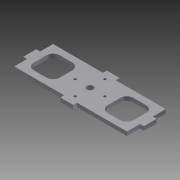
# Autodesk Inventor part: OpenROV 2_2 Horizontal Bulkhead
Saved by Autodesk Inventor 2011 (Build 150239000, 239)
## iProperties
Created: 2011-11-06
Part Number: OpenROV 2_2 Horizontal Bulkhead
Document SubType Name: Modeling
Designer: user
Density: 1 g/cm^3
Author: user
Autodesk Inventor part; units mm, degrees
ref_plane "YZ Plane" through (0, 0, 0) normal (1, 0, 0) x (0, 1, 0)
ref_plane "XZ Plane" through (0, 0, 0) normal (0, 1, 0) x (-1, 0, 0)
ref_plane "XY Plane" through (0, 0, 0) normal (0, 0, 1) x (1, 0, 0)
sketch "Sketch1" plane through (0, 0, 0) normal (0, 0, 1) x (1, 0, 0)
  point P0 (0, 0)
sketch "Sketch2" plane through (0, 0, 0) normal (0, 0, 1) x (1, 0, 0)
  line L0 (0, -10) -> (-3, -10)
  line L1 (-3, -10) -> (-3, -20)
  line L2 (-3, -20) -> (0, -20)
  line L3 (48.5, 0) -> (48.5, 3)
  line L4 (48.5, 3) -> (38.5, 3)
  line L5 (38.5, 3) -> (38.5, 0)
  line L6 (87, -10) -> (90, -10)
  line L7 (90, -10) -> (90, -20)
  line L8 (90, -20) -> (87, -20)
  line L9 (48.5, -30) -> (48.5, -33)
  line L10 (48.5, -33) -> (38.5, -33)
  line L11 (38.5, -33) -> (38.5, -30)
  line L12 (0, 0) -> (38.5, 0)
  line L13 (48.5, 0) -> (87, 0)
  line L14 (0, -30) -> (0, -20)
  line L15 (0, -10) -> (0, 0)
  line L16 (87, -30) -> (48.5, -30)
  line L17 (38.5, -30) -> (0, -30)
  line L18 (87, 0) -> (87, -10)
  line L19 (87, -20) -> (87, -30)
  circle A0 centre (43.5, -15) radius 2.5
  circle A1 centre (43.5, -3.5) radius 1
  line L20 (48.5, 28.5) -> (58.5, 28.5)
  circle A2 centre (32, -15) radius 1
  line L21 (0, -10) -> (0, 0)
  circle A3 centre (43.5, -26.5) radius 1
  line L22 (38.5, -58.5) -> (28.5, -58.5)
  circle A4 centre (55, -15) radius 1
  line L23 (10, -5) -> (20, -5)
  line L24 (25, -10) -> (25, -20)
  line L25 (20, -25) -> (10, -25)
  line L26 (5, -20) -> (5, -10)
  line L27 (67, -5) -> (77, -5)
  line L28 (82, -10) -> (82, -20)
  line L29 (77, -25) -> (67, -25)
  line L30 (62, -20) -> (62, -10)
  arc A5 (10, -5) -> (5, -10) centre (10, -10) ccw
  arc A6 (25, -10) -> (20, -5) centre (20, -10) ccw
  arc A7 (20, -25) -> (25, -20) centre (20, -20) ccw
  arc A8 (5, -20) -> (10, -25) centre (10, -20) ccw
  arc A9 (67, -5) -> (62, -10) centre (67, -10) ccw
  arc A10 (82, -10) -> (77, -5) centre (77, -10) ccw
  arc A11 (77, -25) -> (82, -20) centre (77, -20) ccw
  arc A12 (62, -20) -> (67, -25) centre (67, -20) ccw
  point P0 (5, -5)
  point P1 (25, -5)
  point P2 (62, -5)
  point P3 (82, -5)
  point P4 (62, -25)
  dimension "d0" = 30
  dimension "d1" = 87
  dimension "d2" = 10
  dimension "d3" = 10
  dimension "d4" = 10
  dimension "d5" = 10
  dimension "d6" = 10
  dimension "d7" = 3
  dimension "d8" = 3
  dimension "d9" = 10
  dimension "d10" = 10
  dimension "d11" = 10
  dimension "d12" = 38.5
  dimension "d13" = 38.5
  dimension "d14" = 38.5
  dimension "d15" = 38.5
  dimension "d16" = 3
  dimension "d17" = 3
  dimension "d18" = 3
  dimension "d19" = 3
  dimension "d20" = 3
  dimension "d21" = 5
  dimension "d22" = 2
  dimension "d23" = 11.5
  dimension "d26" = 360
  dimension "d30" = 20
  dimension "d31" = 5
  dimension "d32" = 20
  dimension "d33" = 5
  dimension "d34" = 20
  dimension "d35" = 20
  dimension "d36" = 5
  dimension "d37" = 5
  dimension "d38" = 5
  constraints: 62 end point, 16 parallel, 16 point on circle, 16 tangent, 13 centre point, 10 point on line, 8 perpendicular, 7 equal radius, 6 horizontal, 21 other
  measures "d0" distance of L14.start L12.start
  measures "d1" distance of L12.start L13.end
  measures "d2" distance of L3.end L4.end
  measures "d3" distance of L0.end L1.end
  measures "d4" distance of L9.end L10.end
  measures "d5" distance of L6.end L7.end
  measures "d6" distance of L8.end L16.start
  measures "d7" distance of L7.end L8.end
  measures "d8" distance of L6.start L6.end
  measures "d9" distance of L13.end L6.start
  measures "d10" distance of L14.start L2.end
  measures "d11" distance of L0.start L12.start
  measures "d12" distance of L12.start L5.end
  measures "d13" distance of L11.end L14.start
  measures "d14" distance of L3.start L13.end
  measures "d15" distance of L16.start L9.start
  measures "d16" distance of L9.start L9.end
  measures "d17" distance of L1.end L2.end
  measures "d18" distance of L4.end L5.end
  measures "d19" distance of L3.start L3.end
  measures "d20" distance of L10.end L11.end
  measures "d21" diameter of A0
  measures "d22" diameter of A1
  measures "d23" distance of A0.centre A1.centre
  measures "d30" distance of point (5, -5) point (25, -5)
  measures "d31" distance between parallel lines of L15 L26
  measures "d32" distance between parallel lines of L25 L23
  measures "d33" distance between parallel lines of L12 L23
  measures "d34" distance of point (62, -5) point (82, -5)
  measures "d35" distance of point (62, -25) point (62, -5)
  measures "d36" distance between parallel lines of L18 L28
  measures "d37" distance between parallel lines of L13 L27
  measures "d38" radius of A5
extrude "Extrusion2" add sketch "Sketch2" along normal blind 3
body "Solid2"
